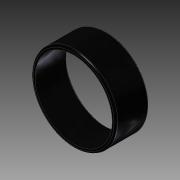
# Autodesk Inventor part: TIRE
Saved by Autodesk Inventor 2014 (Build 180170000, 170)
## iProperties
Created: 2013-10-02
Part Number: TIRE
Material: Generic
Document SubType Name: Modeling
Designer: Brandon
Density: 1 g/cm^3
Appearance: Fine Textured - Black
Author: Brandon
Autodesk Inventor part; units mm, degrees
ref_plane "YZ Plane" through (0, 0, 0) normal (1, 0, 0) x (0, 1, 0)
ref_plane "XZ Plane" through (0, 0, 0) normal (0, 1, 0) x (-1, 0, 0)
ref_plane "XY Plane" through (0, 0, 0) normal (0, 0, 1) x (1, 0, 0)
sketch "Sketch1" plane through (0, 0, 0) normal (0, 0, 1) x (1, 0, 0)
  line L0 (10.5, 0) -> (21, 0) construction
  line L1 (10.5, 0) -> (21, 0) construction
  line L2 (21, 0) -> (21, -0.5)
  line L3 (21, -0.5) -> (20.5, -0.5)
  line L4 (20.5, -0.5) -> (20.5, -8.5)
  line L5 (20.5, -8.5) -> (21.5, -8.5)
  line L6 (21.5, -8.5) -> (21.5, 0)
  line L7 (21.5, 0) -> (21, 0)
  line L8 (10.5, 0) -> (10.5, -8) construction
  line L9 (10.5, 0) -> (18.5, 0) construction
  point P0 (0, 0)
  dimension "d1" = 0
  dimension "d2" = 0.5
  dimension "d3" = 90
  dimension "d4" = 0.5
  dimension "d5" = 270
  dimension "d6" = 8
  dimension "d7" = 1
  dimension "d8" = 8.5
  dimension "d9" = 8
  dimension "d10" = 90
  dimension "d11" = 10.5
  constraints: 20 end point, 4 parallel, 3 horizontal, 3 perpendicular
  measures "d1" distance between parallel lines of L0 L1
  measures "d2" distance of L0.end L2.end
  measures "d3" angle of L0 L2
  measures "d4" distance of L2.end L3.end
  measures "d6" distance of L3.end L4.end
  measures "d7" distance of L4.end L5.end
  measures "d8" distance of L5.end L6.end
  measures "d9" distance of L0.start L8.end
  measures "d10" angle of L8 L9
  measures "d11" distance of L0.start L0.end
revolve "Revolution1" add sketch "Sketch1" angle 360 about axis through (10.5, 0, 0) along (0, -1, 0)
fillet "Fillet1" radius 0.5 1 edges at (-0.5, -8.5, 0)
fillet "Fillet2" radius 0.25 1 edges at (-0.5, 0, 0)
body "Solid1"
